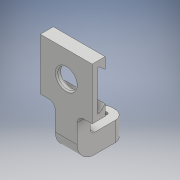
# Autodesk Inventor part: InnerFrame
Saved by Autodesk Inventor 2017 (Build 210142000, 142)
## iProperties
Created: 2016-05-22
Part Number: InnerFrame
Material: Generic
Document SubType Name: Modeling
Designer: Kurtis
Density: 1 g/cm^3
Appearance: Default
Author: Kurtis
Autodesk Inventor part; units mm, degrees
ref_plane "YZ Plane" through (0, 0, 0) normal (1, 0, 0) x (0, 1, 0)
ref_plane "XZ Plane" through (0, 0, 0) normal (0, 1, 0) x (-1, 0, 0)
ref_plane "XY Plane" through (0, 0, 0) normal (0, 0, 1) x (1, 0, 0)
sketch "Sketch1" plane through (0, 0, 0) normal (0, 0, 1) x (1, 0, 0)
  line L0 (-30, -7.5) -> (30, -7.5)
  line L1 (30, -7.5) -> (30, 7.5)
  line L2 (30, 7.5) -> (-30, 7.5)
  line L3 (-30, 7.5) -> (-30, -7.5)
  line L4 (-30, -7.5) -> (30, 7.5) construction
  line L5 (30, -7.5) -> (-30, 7.5) construction
  line L6 (30, 7.5) -> (25, 7.5) construction
  line L7 (-30, 7.5) -> (-25, 7.5) construction
  point P0 (0, 0)
  dimension "d0" = 60
  dimension "d1" = 15
  constraints: 16 end point, 2 midpoint, 2 parallel, 2 point on line, 1 horizontal, 1 perpendicular
  measures "d0" distance of L2.end L1.end
  measures "d1" distance of L1.end L0.end
extrude "Block" add sketch "Sketch1" along normal blind 60
sketch "Sketch2" plane through (30, -7.5, 0) normal (1, 0, 0) x (0, 0, -1)
  line L0 (0, 15) -> (-60, 15) projected
  line L1 (-30, 15) -> (-12.75, 15)
  line L2 (-30, 15) -> (-47.25, 15)
  line L3 (-30, 15) -> (-30, 6.1) construction
  line L4 (-30, 6.1) -> (-6.75, 6.1)
  line L5 (-30, 6.1) -> (-53.25, 6.1)
  line L6 (-53.25, 6.1) -> (-53.25, 8.1)
  line L7 (-6.75, 6.1) -> (-6.75, 8.1)
  line L8 (-6.75, 8.1) -> (-12.75, 15)
  line L9 (-53.25, 8.1) -> (-47.25, 15)
  point P0 (0, 7.5)
  dimension "d17" = 17.25
  dimension "d18" = 17.25
  dimension "d19" = 8.9
  dimension "d20" = 23.25
  dimension "d21" = 23.25
  dimension "d22" = 2
  dimension "d23" = 2
  constraints: 18 end point, 2 perpendicular, 2 point on line, 2 vertical, 1 horizontal, 1 midpoint
  measures "d17" distance of L1.start L1.end
  measures "d18" distance of L1.start L2.end
  measures "d19" distance of L1.start L3.end
  measures "d20" distance of L3.end L4.end
  measures "d21" distance of L3.end L5.end
  measures "d22" distance of L5.end L6.end
  measures "d23" distance of L4.end L7.end
extrude "Tripod Slot" cut sketch "Sketch2" against normal blind 60
hole "Hole1" at (0, -1.4, 30) direction (0, -1, 0) diameter 22.5 end through all
sketch "Sketch4" plane through (0, 0, 0) normal (0, 0, -1) x (-1, 0, 0)
  line L0 (-30, 7.5) -> (30, 7.5) projected
  line L1 (12.7, 7.5) -> (-12.7, 7.5)
  line L2 (-12.7, 7.5) -> (-12.7, -7.5)
  line L3 (30, -7.5) -> (-30, -7.5) projected
  line L4 (-12.7, -7.5) -> (12.7, -7.5)
  line L5 (12.7, -7.5) -> (12.7, 7.5)
  point P0 (0, 1.5)
  dimension "d64" = 25.4
  dimension "d96" = 17.3
  dimension "d97" = 9
  dimension "d98" = 12.7
  constraints: 8 end point, 2 point on line, 1 horizontal, 1 parallel, 1 perpendicular, 1 vertical
  measures "d64" distance of L1.end L1.start
  measures "d96" distance from line of L0.end L5
  measures "d97" distance from line of point (0, 1.5) L3
  measures "d98" distance from line of point (0, 1.5) L5
extrude "Extrusion4" add sketch "Sketch4" along normal blind 49.5
sketch "Sketch5" plane through (-30, 7.5, 12.75) normal (0, 1, 0) x (1, 0, 0)
  line L0 (60, -34.5) -> (60, 0) projected
  line L1 (17.3, 62.25) -> (42.7, 62.25) projected
  line L2 (17.3, 62.25) -> (42.7, 62.25)
  line L3 (42.7, 62.25) -> (42.7, 39.75)
  line L4 (42.7, 39.75) -> (17.3, 39.75)
  line L5 (17.3, 39.75) -> (17.3, 62.25)
  line L6 (42.7, 39.75) -> (17.3, 62.25) construction
  circle A0 centre (30, 51) radius 1.5
  point P0 (30, 12.75)
  dimension "d67" = 22.5
  dimension "d68" = 3
  dimension "d99" = 131.535
  constraints: 10 end point, 2 parallel, 1 centre point, 1 horizontal, 1 midpoint, 1 perpendicular
  measures "d67" distance of L2.end L3.end
  measures "d68" diameter of A0
  measures "d99" angle of L0 L6
extrude "Extrusion5" add sketch "Sketch5" along normal blind 40
sketch "Sketch6" plane through (0, 0, -49.5) normal (0, 0, -1) x (-1, 0, 0)
  line L0 (0, 0) -> (0, 47.5) construction
  circle A0 centre (0, 37.5) radius 2.5
  line L1 (-12.7, 47.5) -> (12.7, 47.5) construction
  line L2 (-12.7, 47.5) -> (12.7, 47.5) construction
  line L3 (12.7, 47.5) -> (0, 47.5) construction
  line L4 (0, 37.5) -> (0, 47.5) construction
  dimension "d60" = 5
  dimension "d61" = 10
  constraints: 8 end point, 3 collinear, 1 centre point, 1 point on line
  measures "d60" diameter of A0
  measures "d61" distance of L0.end L4.start
extrude "Extrusion6" cut sketch "Sketch6" against normal blind 31.75
fillet "Fillet4" radius 11 2 edges at (12.7, 47.5, -38.25) (-12.7, 47.5, -38.25)
fillet "Fillet5" radius 20 1 edges at (0, -7.5, -49.5)
fillet "Fillet6" radius 5 1 edges at (0, 7.5, -27)
fillet "Fillet10" radius 7.5 2 edges at (12.7, 0, 0) (-12.7, 0, 0)
fillet "Fillet11" radius 1.5 2 edges at (0, -7.5, 18.75) (0, -1.4, 18.75)
body "Solid1"
